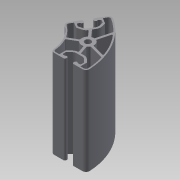
# Autodesk Inventor part: 40-4096
Saved by Autodesk Inventor 2013 (Build 170138000, 138)
## iProperties
Created: 2014-04-23
Part Number: 40-4096
Material: Generic
Document SubType Name: Modeling
Designer: Ross Bowman
Density: 1 g/cm^3
Engineer: Ross Bowman
Catalog Web Link: 8020.net
Vendor: 80/20 Inc.
Company: 80/20 Inc.
Author: Ross Bowman
Keywords: 80/20 , 8020 , T-Slot , Extrusion
Material: 6105-T5 Aluminum
Autodesk Inventor part; units mm, degrees
ref_plane "YZ Plane" through (0, 0, 0) normal (1, 0, 0) x (0, 1, 0)
ref_plane "XZ Plane" through (0, 0, 0) normal (0, 1, 0) x (-1, 0, 0)
ref_plane "XY Plane" through (0, 0, 0) normal (0, 0, 1) x (1, 0, 0)
sketch "Sketch1" plane through (0, 0, 0) normal (0, 0, 1) x (1, 0, 0)
  circle A0 centre (0, 0) radius 3.3782
  arc A1 (7.4032, -15.0221) -> (8.0031, -15.4492) centre (8.0031, -14.8142) ccw
  line L0 (4.2986, -6.0652) -> (7.4032, -15.0221)
  arc A2 (4.4912, -5.3702) -> (4.2986, -6.0652) centre (4.8985, -5.8573) ccw
  arc A3 (4.4912, -5.3702) -> (6.0273, -3.5609) centre (0.0003, -0.0006) ccw
  arc A4 (6.7358, -3.2699) -> (6.0273, -3.5609) centre (6.574, -3.8839) ccw
  line L1 (22.6399, -7.4601) -> (6.7358, -3.2699)
  arc A5 (23.1755, -7.981) -> (22.6399, -7.4601) centre (22.4462, -8.195) ccw
  arc A6 (26.2424, -25.9962) -> (23.1755, -7.981) centre (-52.0623, -30.0582) ccw
  arc A7 (23.8956, -28.468) -> (26.2424, -25.9962) centre (23.8956, -26.118) ccw
  line L2 (20.592, -28.468) -> (23.8956, -28.468)
  arc A8 (19.957, -27.833) -> (20.592, -28.468) centre (20.592, -27.833) ccw
  line L3 (19.957, -21.3543) -> (19.957, -27.833)
  arc A9 (19.957, -21.3543) -> (19.7702, -20.9031) centre (19.319, -21.3543) ccw
  line L4 (16.3781, -17.5111) -> (19.7702, -20.9031)
  arc A10 (16.3781, -17.5111) -> (11.4002, -15.4492) centre (11.4002, -22.489) ccw
  line L5 (8.0031, -15.4492) -> (11.4002, -15.4492)
  arc A11 (2.0629, -7.2835) -> (1.3421, -6.8708) centre (1.4638, -7.494) ccw
  line L6 (4.6432, -14.6255) -> (2.0629, -7.2835)
  arc A12 (4.0921, -15.4692) -> (4.6432, -14.6255) centre (4.0441, -14.836) ccw
  arc A13 (4.0921, -15.4692) -> (-0.3284, -17.4994) centre (4.6214, -22.4492) ccw
  line L7 (-3.7321, -20.9031) -> (-0.3284, -17.4994)
  arc A14 (-3.7321, -20.9031) -> (-3.919, -21.3543) centre (-3.281, -21.3543) ccw
  line L8 (-3.919, -27.833) -> (-3.919, -21.3543)
  arc A15 (-4.554, -28.468) -> (-3.919, -27.833) centre (-4.554, -27.833) ccw
  line L9 (-8.3232, -28.468) -> (-4.554, -28.468)
  arc A16 (-10.6638, -26.3288) -> (-8.3232, -28.468) centre (-8.3232, -26.118) ccw
  arc A17 (-10.6638, -26.3288) -> (-15.1632, -10.9217) centre (-52.0623, -30.0582) ccw
  arc A18 (-14.917, -10.0795) -> (-15.1632, -10.9217) centre (-14.5995, -10.6294) ccw
  line L10 (-5.7677, -4.7972) -> (-14.917, -10.0795)
  arc A19 (-4.9969, -4.9024) -> (-5.7677, -4.7972) centre (-5.4502, -5.3471) ccw
  arc A20 (-4.9969, -4.9024) -> (1.3421, -6.8708) centre (0.0003, -0.0006) ccw
  arc A21 (-20.4627, 7.2657) -> (-19.9786, 7.2019) centre (-20.1437, 7.8182) ccw
  line L11 (-15.3291, 8.4478) -> (-19.9786, 7.2019)
  arc A22 (-15.3291, 8.4478) -> (-11.3505, 11.2757) centre (-17.1408, 15.2093) ccw
  arc A23 (-10.3434, 11.3324) -> (-11.3505, 11.2757) centre (-10.8253, 10.9189) ccw
  line L12 (-5.2755, 5.4271) -> (-10.3434, 11.3324)
  arc A24 (-5.2785, 4.5966) -> (-5.2755, 5.4271) centre (-5.7574, 5.0136) ccw
  arc A25 (-5.2785, 4.5966) -> (-6.7434, -1.8773) centre (0.0003, -0.0006) ccw
  arc A26 (-7.0377, -2.5975) -> (-6.7434, -1.8773) centre (-7.3552, -2.0475) ccw
  line L13 (-16.187, -7.8797) -> (-7.0377, -2.5975)
  arc A27 (-17.0395, -7.6718) -> (-16.187, -7.8797) centre (-16.5045, -7.3298) ccw
  arc A28 (-17.0395, -7.6718) -> (-28.0922, 3.9004) centre (-52.0623, -30.0582) ccw
  arc A29 (-28.7595, 7.0169) -> (-28.0922, 3.9004) centre (-26.737, 5.8203) ccw
  line L14 (-26.8571, 10.2321) -> (-28.7595, 7.0169)
  arc A30 (-25.9931, 10.4587) -> (-26.8571, 10.2321) centre (-26.3106, 9.9087) ccw
  line L15 (-20.4627, 7.2657) -> (-25.9931, 10.4587)
  arc A31 (21.6555, -3.3409) -> (7.9566, 20.3984) centre (-52.0623, -30.0582) ccw
  arc A32 (20.7474, -4.3348) -> (21.6555, -3.3409) centre (20.941, -3.5999) ccw
  line L16 (7.4703, -0.8367) -> (20.7474, -4.3348)
  arc A33 (6.9974, -0.2042) -> (7.4703, -0.8367) centre (7.6321, -0.2227) ccw
  arc A34 (6.9974, -0.2042) -> (3.3247, 6.1597) centre (0.0003, -0.0006) ccw
  arc A35 (3.0139, 6.8865) -> (3.3247, 6.1597) centre (3.6263, 6.7185) ccw
  line L17 (6.6419, 20.1104) -> (3.0139, 6.8865)
  arc A36 (7.9566, 20.3984) -> (6.6419, 20.1104) centre (7.3748, 19.9093) ccw
  arc A37 (4.7026, 24.0332) -> (-9.3424, 35.6924) centre (-52.0623, -30.0582) ccw
  arc A38 (4.8853, 23.3078) -> (4.7026, 24.0332) centre (4.1524, 23.5089) ccw
  line L18 (0.539, 7.4661) -> (4.8853, 23.3078)
  arc A39 (-0.0672, 6.9991) -> (0.539, 7.4661) centre (-0.0733, 7.6341) ccw
  arc A40 (-0.0672, 6.9991) -> (-2.4044, 6.5734) centre (0.0003, -0.0006) ccw
  arc A41 (-3.1026, 6.7541) -> (-2.4044, 6.5734) centre (-2.6225, 7.1698) ccw
  line L19 (-9.3079, 13.9221) -> (-3.1026, 6.7541)
  arc A42 (-9.3777, 14.6553) -> (-9.3079, 13.9221) centre (-8.8278, 14.3378) ccw
  line L20 (-7.6892, 17.58) -> (-9.3777, 14.6553)
  arc A43 (-7.6892, 17.58) -> (-6.9859, 22.9219) centre (-13.7858, 21.0999) ccw
  line L21 (-8.2275, 27.5555) -> (-6.9859, 22.9219)
  arc A44 (-8.2275, 27.5555) -> (-8.5247, 27.9429) centre (-8.8437, 27.3904) ccw
  line L22 (-14.0551, 31.1359) -> (-8.5247, 27.9429)
  arc A45 (-14.2909, 31.9974) -> (-14.0551, 31.1359) centre (-13.7376, 31.6858) ccw
  line L23 (-12.6703, 34.875) -> (-14.2909, 31.9974)
  arc A46 (-9.3424, 35.6924) -> (-12.6703, 34.875) centre (-10.6227, 33.7218) ccw
  arc A47 (12.0825, -28.4745) -> (13.5936, -30.058) centre (13.6759, -28.4667) ccw
  line L24 (13.5936, -30.058) -> (23.8323, -30.058)
  arc A48 (23.8323, -30.058) -> (27.8268, -25.8474) centre (23.8323, -26.058) ccw
  arc A49 (27.8268, -25.8474) -> (-8.4712, 37.0225) centre (-52.0623, -30.0582) ccw
  arc A50 (-8.4712, 37.0225) -> (-14.1148, 35.6684) centre (-10.6507, 33.6684) ccw
  line L25 (-14.1148, 35.6684) -> (-19.2342, 26.8014)
  arc A51 (-19.2342, 26.8014) -> (-18.6184, 24.701) centre (-17.815, 26.077) ccw
  line L26 (-18.6184, 24.701) -> (-17.8266, 24.2438)
  arc A52 (-17.8266, 24.2438) -> (-15.7151, 24.7696) centre (-17.0413, 25.5926) ccw
  line L27 (-15.7151, 24.7696) -> (-15.3301, 25.4365)
  arc A53 (-15.3301, 25.4365) -> (-15.4578, 25.9486) centre (-15.6592, 25.6264) ccw
  line L28 (-15.4578, 25.9486) -> (-15.482, 25.9638)
  arc A54 (-15.6097, 26.476) -> (-15.482, 25.9638) centre (-15.2807, 26.286) ccw
  line L29 (-15.6097, 26.476) -> (-14.6543, 28.1308)
  arc A55 (-12.9197, 28.5956) -> (-14.6543, 28.1308) centre (-13.5546, 27.4959) ccw
  line L30 (-12.9197, 28.5956) -> (-10.8065, 27.3756)
  arc A56 (-10.3923, 26.8358) -> (-10.8065, 27.3756) centre (-11.2509, 26.6058) ccw
  line L31 (-10.3923, 26.8358) -> (-9.1894, 22.3466)
  arc A57 (-9.6639, 18.7428) -> (-9.1894, 22.3466) centre (-13.7768, 21.1174) ccw
  line L32 (-9.6639, 18.7428) -> (-13.0446, 12.8871)
  arc A58 (-15.9284, 10.6743) -> (-13.0446, 12.8871) centre (-17.1576, 15.2617) ccw
  line L33 (-15.9284, 10.6743) -> (-20.4177, 9.4714)
  arc A59 (-21.0922, 9.5602) -> (-20.4177, 9.4714) centre (-20.6477, 10.33) ccw
  line L34 (-21.0922, 9.5602) -> (-23.2053, 10.7802)
  arc A60 (-23.6701, 12.5149) -> (-23.2053, 10.7802) centre (-22.5704, 11.8799) ccw
  line L35 (-23.6701, 12.5149) -> (-22.7147, 14.1697)
  arc A61 (-22.2073, 14.3152) -> (-22.7147, 14.1697) centre (-22.3857, 13.9797) ccw
  line L36 (-22.2073, 14.3152) -> (-22.1821, 14.3018)
  arc A62 (-22.1821, 14.3018) -> (-21.6747, 14.4473) centre (-22.0037, 14.6373) ccw
  line L37 (-21.6747, 14.4473) -> (-21.3214, 15.0591)
  arc A63 (-21.3214, 15.0591) -> (-21.8978, 17.2101) centre (-22.6851, 15.8464) ccw
  line L38 (-21.8978, 17.2101) -> (-22.6896, 17.6672)
  arc A64 (-22.6896, 17.6672) -> (-24.8405, 17.0909) centre (-23.4769, 16.3036) ccw
  line L39 (-24.8405, 17.0909) -> (-30.1429, 7.9069)
  arc A65 (-30.1429, 7.9069) -> (-28.9846, 2.6383) centre (-26.6788, 5.9069) ccw
  arc A66 (-12.2074, -26.4206) -> (-28.9846, 2.6383) centre (-52.0426, -30.0469) ccw
  arc A67 (-12.2074, -26.4206) -> (-8.2238, -30.058) centre (-8.2238, -26.058) ccw
  line L40 (-8.2238, -30.058) -> (2.3809, -30.058)
  arc A68 (2.3809, -30.058) -> (3.9555, -28.4834) centre (2.3809, -28.4834) ccw
  line L41 (3.9555, -28.4834) -> (3.9555, -27.5691)
  arc A69 (3.9555, -27.5691) -> (2.3809, -25.9945) centre (2.3809, -27.5691) ccw
  line L42 (2.3809, -25.9945) -> (1.6745, -25.9945)
  arc A70 (1.6745, -25.9945) -> (1.2947, -26.3612) centre (1.6745, -26.3744) ccw
  line L43 (1.2947, -26.3612) -> (1.2937, -26.3897)
  arc A71 (0.914, -26.7564) -> (1.2937, -26.3897) centre (0.914, -26.3764) ccw
  line L44 (0.914, -26.7564) -> (-0.9968, -26.7564)
  arc A72 (-2.2667, -25.4865) -> (-0.9968, -26.7564) centre (-0.9968, -25.4865) ccw
  line L45 (-2.2667, -25.4865) -> (-2.2667, -23.0464)
  arc A73 (-2.0063, -22.4179) -> (-2.2667, -23.0464) centre (-1.3778, -23.0464) ccw
  line L46 (-2.0063, -22.4179) -> (1.2801, -19.1315)
  arc A74 (4.6383, -17.7405) -> (1.2801, -19.1315) centre (4.6383, -22.4897) ccw
  line L47 (4.6383, -17.7405) -> (11.3998, -17.7405)
  arc A75 (14.758, -19.1315) -> (11.3998, -17.7405) centre (11.3998, -22.4897) ccw
  line L48 (14.758, -19.1315) -> (18.0444, -22.4179)
  arc A76 (18.3048, -23.0464) -> (18.0444, -22.4179) centre (17.4159, -23.0464) ccw
  line L49 (18.3048, -23.0464) -> (18.3048, -25.4865)
  arc A77 (17.0349, -26.7564) -> (18.3048, -25.4865) centre (17.0349, -25.4865) ccw
  line L50 (17.0349, -26.7564) -> (15.124, -26.7564)
  arc A78 (14.7443, -26.3897) -> (15.124, -26.7564) centre (15.124, -26.3764) ccw
  line L51 (14.7443, -26.3897) -> (14.7433, -26.3612)
  arc A79 (14.7433, -26.3612) -> (14.3636, -25.9945) centre (14.3636, -26.3744) ccw
  line L52 (14.3636, -25.9945) -> (13.5936, -25.9945)
  arc A80 (13.5936, -25.9945) -> (12.0825, -27.5602) centre (13.6433, -27.5544) ccw
  line L53 (12.0825, -27.5602) -> (12.0825, -28.4745)
  constraints: 160 point on circle, 108 end point, 81 centre point
extrude "Extrusion1" add sketch "Sketch1" against normal blind 100
body "Solid1"
